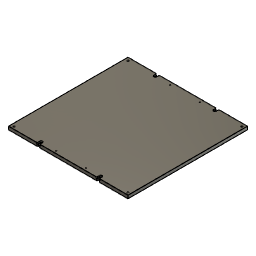
Voron_V2.4_300x300_BuildPlate (Autodesk Fusion 360 design; units mm, degrees)
Autodesk Fusion 360 part; units mm, degrees
sketch "Sketch1" plane through (0, 0, 0) normal (0, 1, 0) x (1, 0, 0)
  line L0 (0, 0) -> (300.8, 0)
  line L1 (300.8, 0) -> (300.8, 300.8)
  line L2 (300.8, 300.8) -> (0, 300.8)
  line L3 (0, 300.8) -> (0, 0)
  line L4 (0, 0) -> (7, 0)
  line L5 (7, 0) -> (7, 7) construction
  line L6 (7, 7) -> (0, 7) construction
  line L7 (0, 7) -> (0, 0)
  circle A0 centre (7, 7) radius 2.1
  line L8 (300.8, 0) -> (293.8, 0)
  line L9 (293.8, 0) -> (293.8, 7) construction
  line L10 (293.8, 7) -> (300.8, 7) construction
  line L11 (300.8, 7) -> (300.8, 0)
  circle A1 centre (293.8, 7) radius 2.1
  line L12 (150.4, 0) -> (150.4, 7) construction
  line L13 (150.4, 7) -> (75.4, 7) construction
  circle A2 centre (75.4, 7) radius 1.7
  circle A3 centre (75.4, 7) radius 3.25
  circle A4 centre (225.4, 7) radius 3.25
  circle A5 centre (225.4, 7) radius 1.7
  line L14 (300.8, 150.4) -> (290.8, 150.4) construction
  circle A6 centre (225.4, 293.8) radius 3.25
  circle A7 centre (225.4, 293.8) radius 1.7
  circle A8 centre (75.4, 293.8) radius 3.25
  circle A9 centre (75.4, 293.8) radius 1.7
  dimension "d1" = 300.8
  dimension "d2" = 300.8
  dimension "d3" = 7
  dimension "d4" = 7
  dimension "d5" = 4.2
  dimension "d6" = 7
  dimension "d7" = 7
  dimension "d8" = 4.2
  dimension "d9" = 7
  dimension "d10" = 75
  dimension "d11" = 3.4
  dimension "d12" = 6.5
  dimension "d13" = 10
  constraint horizontal L0
  constraint vertical L1
  constraint horizontal L2
  constraint vertical L3
  constraint coincident L0.start L3.end
  constraint horizontal L4
  constraint vertical L5
  constraint horizontal L6
  constraint vertical L7
  constraint coincident L5.end L6.start
  constraint horizontal L8
  constraint vertical L9
  constraint horizontal L10
  constraint vertical L11
  constraint coincident L9.end L10.start
  constraint midpoint L0 L12.start
  constraint vertical L12
  constraint perpendicular L12 L13
  constraint coincident L13.end A2.centre
  constraint concentric A2 A3
  constraint symmetric L12 A2 A5
  constraint symmetric L12 A3 A4
  constraint midpoint L1 L14.start
  constraint horizontal L14
  constraint symmetric A2 L14 A9
  constraint symmetric A3 L14 A8
  constraint symmetric A4 L14 A6
  constraint symmetric A5 L14 A7
  measures "d1" distance of L0.start L0.end
  measures "d2" distance of L0.start L2.end
  measures "d3" distance of L0.start L4.end
  measures "d4" distance of L0.start L6.end
  measures "d5" diameter of A0
  measures "d6" distance of L0.end L8.end
  measures "d7" distance of L0.end L10.end
  measures "d8" diameter of A1
  measures "d9" distance of L12.start L12.end
  measures "d10" distance of L12.end L13.end
  measures "d11" diameter of A2
  measures "d12" diameter of A3
  measures "d13" distance of L14.start L14.end
extrude "Extrude1" add sketch "Sketch1" along normal blind 8 contours L0 L1 L2 L3 L4 L7 L8 L11 | A0 | A1 | A3 | A4 | A6 | A8 makes body 1
extrude "Extrude2" cut sketch "Sketch1" along normal blind 6 contours A0 | A1 bodies 1
extrude "Extrude3" cut sketch "Sketch1" along normal blind 75 and the other way blind -4.5 contours A3 | A4 | A6 | A8 bodies 1
copy_body "Body->Comp1" bodies 1 removing the originals makes body 2 in component "Component"
chamfer "Chamfer1" distance 0.2 angle 45 8 edges at (300.8, 8, -150.4) (150.4, 8, 0) (0, 8, -150.4) (150.4, 8, -300.8) (0, 0, -150.4) (150.4, 0, 0) (300.8, 0, -150.4) (150.4, 0, -300.8) on bodies 2 in component "Component"
fillet "Fillet1" radius 0.2 4 edges at (300.8, 4, -300.8) (0, 4, -300.8) (0, 4, 0) (300.8, 4, 0) on bodies 2 in component "Component"
thread "Thread1" "ISO Metric profile 5.0 M5x0.8 6H" major diameter 5.12 minor diameter 4.234 pitch 0.8 angle 60 resizes the face on face at (9.0974, 4, -6.8953) on face at (294.6637, 4, -8.9142) on bodies 2 in component "Component"
delete_face "DeleteFace1" 1 faces at (300.7333, 7.8667, -200.4667) on bodies 2 in component "Component"
delete_face "DeleteFace2" 1 faces at (200.5333, 7.9333, -0.1333) on bodies 2 in component "Component"
delete_face "DeleteFace3" 1 faces at (200.4667, 0.1333, -0.0667) on bodies 2 in component "Component"
delete_face "DeleteFace4" 1 faces at (300.6667, 0.0667, -100.2667) on bodies 2 in component "Component"
delete_face "DeleteFace5" 1 faces at (200.5333, 0.0667, -300.6667) on bodies 2 in component "Component"
delete_face "DeleteFace6" 1 faces at (200.5333, 7.9333, -300.6667) on bodies 2 in component "Component"
delete_face "DeleteFace7" 1 faces at (0.1333, 7.9333, -200.4667) on bodies 2 in component "Component"
delete_face "DeleteFace8" 1 faces at (0.1333, 0.0667, -100.3333) on bodies 2 in component "Component"
delete_face "DeleteFace9" 1 faces at (295.0358, 4, -8.7189) on bodies 2 in component "Component"
delete_face "DeleteFace10" 1 faces at (9.1144, 2, -7.1055) on bodies 2 in component "Component"
sketch "Sketch3" plane through (0, 8, 0) normal (0, 1, 0) x (-1, 0, 0)
  circle A0 centre (-75.4, -293.8) radius 3.25
  circle A1 centre (-225.4, -7) radius 3.25
  circle A2 centre (-225.4, -293.8) radius 3.25
  circle A3 centre (-75.4, -7) radius 3.25
  arc A4 (0, -0.2) -> (-0.2, 0) centre (-0.2, -0.2) ccw
  line L0 (-0.2, 0) -> (-300.6, 0)
  arc A5 (-300.6, 0) -> (-300.8, -0.2) centre (-300.6, -0.2) ccw
  line L1 (-300.8, -0.2) -> (-300.8, -300.6)
  arc A6 (-300.8, -300.6) -> (-300.6, -300.8) centre (-300.6, -300.6) ccw
  line L2 (-300.6, -300.8) -> (-0.2, -300.8)
  arc A7 (-0.2, -300.8) -> (0, -300.6) centre (-0.2, -300.6) ccw
  line L3 (0, -300.6) -> (0, -0.2)
  line L4 (-225.4, -7) -> (-228.65, -7) construction
  line L5 (-225.4, -7) -> (-222.15, -7) construction
  line L6 (-228.65, -7) -> (-228.65, 0)
  line L7 (-222.15, -7) -> (-222.15, 0)
  constraint coincident A1.centre L4.start
  constraint coincident A1 L4.end
  constraint horizontal L4
  constraint coincident A1 L5.end
  constraint parallel L4 L5
  constraint coincident L0 L6.end
  constraint tangent A1 L6
  constraint coincident L0 L7.end
  constraint tangent A1 L7
extrude "Extrude1'" cut sketch "Sketch3" against normal blind 3.5 contours A1 L0 L6 L7 bodies 2 in component "Component"
sketch "Sketch4" plane through (0, 4.5, 0) normal (0, 1, 0) x (-1, 0, 0)
  circle A0 centre (-225.4, -7) radius 1.7
  arc A1 (-228.65, -7) -> (-222.15, -7) centre (-225.4, -7) ccw
  line L0 (-222.15, -7) -> (-222.15, 0)
  line L1 (-222.15, 0) -> (-228.65, 0)
  line L2 (-228.65, 0) -> (-228.65, -7)
  line L3 (-225.4, -7) -> (-227.1, -7) construction
  line L4 (-225.4, -7) -> (-223.7, -7) construction
  line L5 (-227.1, -7) -> (-227.1, 0)
  line L6 (-223.7, -7) -> (-223.7, 0)
  constraint coincident A0.centre A1.centre
  constraint coincident A0 L3.end
  constraint horizontal L3
  constraint coincident A0 L4.end
  constraint horizontal L4
  constraint coincident L1 L5.end
  constraint tangent A0 L5
  constraint coincident L1 L6.end
  constraint tangent A0 L6
extrude "Extrude2'" cut sketch "Sketch4" against normal blind 12 contours A0 L1 L5 L6 bodies 2 in component "Component"
fillet "Fillet2" radius 2 4 edges at (228.65, 6.25, 0) (227.1, 2.25, 0) (223.7, 2.25, 0) (222.15, 6.25, 0) on bodies 2 in component "Component"
ref_plane "WorkPlane1" through (110.95, 4, -150.4) normal (0, 0, 1) x (1, 0, 0)
mirror "Mirror1" about plane through (110.95, 4, -150.4) normal (0, 0, 1) of 11 faces at (230.1785, 6.8333, -0.0564) (228.65, 5.6667, -3.6667) (228.6339, 6.8333, -7.3236) (222.6667, 4.5, -5.3333) (223.7084, 1.5, -7.1693) (227.1, 3, -5.3333) (228.9099, 1.5, -0.0091) (222.0785, 1.5, -0.0361) (223.7, 3, -5.3333) (222.15, 6.8333, -5.3333) (220.6215, 5.6667, -0.0564) on bodies 2 in component "Component"
ref_plane "WorkPlane2" through (150.4, 4, -150.4) normal (1, 0, 0) x (0, 0, -1)
mirror "Mirror2" about plane through (150.4, 4, -150.4) normal (1, 0, 0) of 22 faces at (220.6215, 5.6667, -0.0564) (222.15, 6.8333, -5.3333) (228.6339, 6.8333, -7.3236) (222.6667, 4.5, -5.3333) (222.0785, 1.5, -0.0361) (223.7, 3, -5.3333) (223.7084, 1.5, -7.1693) (227.1, 3, -5.3333) (228.9099, 1.5, -0.0091) (228.65, 5.6667, -3.6667) (230.1785, 6.8333, -0.0564) (222.0785, 1.5, -300.7639) (223.7, 3, -295.4667) (223.7526, 3, -293.3805) (222.4052, 6.8333, -292.5376) (222.15, 6.8333, -295.4667) (220.6215, 5.6667, -300.7436) (222.6667, 4.5, -295.4667) (228.9099, 1.5, -300.7909) (227.1, 3, -295.4667) (228.65, 6.8333, -295.4667) (230.2715, 5.6667, -300.7639) on bodies 2 in component "Component"
chamfer "Chamfer4" distance 0.2 angle 45 64 edges at (221.5642, 8, -0.5858) (222.15, 8, -4.5) (225.4, 8, -10.25) (228.65, 8, -4.5) (229.2358, 8, -0.5858) (265.625, 8, 0) (300.7414, 8, -0.0586) (300.8, 8, -150.4) (300.7414, 8, -300.7414) (265.625, 8, -300.8) (229.2358, 8, -300.2142) (228.65, 8, -296.3) (225.4, 8, -290.55) (222.15, 8, -296.3) (221.5642, 8, -300.2142) (150.4, 8, -300.8) (79.2358, 8, -300.2142) (78.65, 8, -296.3) (75.4, 8, -290.55) (72.15, 8, -296.3) (71.5642, 8, -300.2142) (35.175, 8, -300.8) (0.0586, 8, -300.7414) (0, 8, -150.4) (0.0586, 8, -0.0586) (35.175, 8, 0) (71.5642, 8, -0.5858) (72.15, 8, -4.5) (75.4, 8, -10.25) (78.65, 8, -4.5) (79.2358, 8, -0.5858) (150.4, 8, 0) (77.6858, 0, -0.5858) (77.1, 0, -4.5) (75.4, 0, -8.7) (73.7, 0, -4.5) (73.1142, 0, -0.5858) (35.95, 0, 0) (0.0586, 0, -0.0586) (0, 0, -150.4) (0.0586, 0, -300.7414) (35.95, 0, -300.8) (73.1142, 0, -300.2142) (73.7, 0, -296.3) (75.4, 0, -292.1) (77.1, 0, -296.3) (77.6858, 0, -300.2142) (150.4, 0, -300.8) (223.1142, 0, -300.2142) (223.7, 0, -296.3) (225.4, 0, -292.1) (227.1, 0, -296.3) (227.6858, 0, -300.2142) (264.85, 0, -300.8) (300.7414, 0, -300.7414) (300.8, 0, -150.4) (300.7414, 0, -0.0586) (264.85, 0, 0) (227.6858, 0, -0.5858) (227.1, 0, -4.5) (225.4, 0, -8.7) (223.7, 0, -4.5) (223.1142, 0, -0.5858) (150.4, 0, 0) on bodies 2 in component "Component"
sketch "Sketch5" plane through (0, 0, 0) normal (0, -1, 0) x (1, 0, 0)
  arc A0 (79.1, -0.2) -> (77.3, -2) centre (79.1, -2) ccw
  line L0 (77.3, -2) -> (77.3, -7)
  arc A1 (73.5, -7) -> (77.3, -7) centre (75.4, -7) ccw
  line L1 (73.5, -7) -> (73.5, -2)
  arc A2 (73.5, -2) -> (71.7, -0.2) centre (71.7, -2) ccw
  line L2 (71.7, -0.2) -> (0.2, -0.2)
  line L3 (0.2, -0.2) -> (0.2, -300.6)
  line L4 (0.2, -300.6) -> (71.7, -300.6)
  arc A3 (71.7, -300.6) -> (73.5, -298.8) centre (71.7, -298.8) ccw
  line L5 (73.5, -298.8) -> (73.5, -293.8)
  arc A4 (77.3, -293.8) -> (73.5, -293.8) centre (75.4, -293.8) ccw
  line L6 (77.3, -293.8) -> (77.3, -298.8)
  arc A5 (77.3, -298.8) -> (79.1, -300.6) centre (79.1, -298.8) ccw
  line L7 (79.1, -300.6) -> (221.7, -300.6)
  arc A6 (221.7, -300.6) -> (223.5, -298.8) centre (221.7, -298.8) ccw
  line L8 (223.5, -298.8) -> (223.5, -293.8)
  arc A7 (227.3, -293.8) -> (223.5, -293.8) centre (225.4, -293.8) ccw
  line L9 (227.3, -293.8) -> (227.3, -298.8)
  arc A8 (227.3, -298.8) -> (229.1, -300.6) centre (229.1, -298.8) ccw
  line L10 (229.1, -300.6) -> (300.6, -300.6)
  line L11 (300.6, -300.6) -> (300.6, -0.2)
  line L12 (300.6, -0.2) -> (229.1, -0.2)
  arc A9 (229.1, -0.2) -> (227.3, -2) centre (229.1, -2) ccw
  line L13 (227.3, -2) -> (227.3, -7)
  arc A10 (223.5, -7) -> (227.3, -7) centre (225.4, -7) ccw
  line L14 (223.5, -7) -> (223.5, -2)
  arc A11 (223.5, -2) -> (221.7, -0.2) centre (221.7, -2) ccw
  line L15 (221.7, -0.2) -> (79.1, -0.2)
  line L16 (0, -0.2) -> (0, -300.6)
  line L17 (0.2, -300.8) -> (71.7, -300.8)
  line L18 (0, -293.8) -> (7, -293.8) construction
  line L19 (7, -293.8) -> (7, -300.8) construction
  circle A12 centre (7, -293.8) radius 2.1
  line L20 (79.1, -300.8) -> (221.7, -300.8)
  line L21 (150.4, -300.8) -> (150.4, 0) construction
  line L22 (150.4, -300.8) -> (150.4, -293.8) construction
  line L23 (150.4, -293.8) -> (112.9, -293.8) construction
  circle A13 centre (112.9, -293.8) radius 1.25
  circle A14 centre (293.8, -293.8) radius 2.1
  circle A15 centre (187.9, -293.8) radius 1.25
  line L24 (79.1, -0.2) -> (221.7, -0.2)
  line L25 (221.7, 0) -> (79.1, 0)
  line L26 (150.4, -150.4) -> (231.0911, -150.4) construction
  circle A16 centre (7, -7) radius 2.1
  circle A17 centre (112.9, -7) radius 1.25
  circle A18 centre (187.9, -7) radius 1.25
  circle A19 centre (293.8, -7) radius 2.1
  dimension "d36" = 7
  dimension "d37" = 7
  dimension "d38" = 4.2
  dimension "d39" = 7
  dimension "d40" = 37.5
  dimension "d41" = 2.5
  constraint coincident L16 L18.start
  constraint perpendicular L3 L18
  constraint coincident L17 L19.end
  constraint perpendicular L17 L19
  constraint coincident L18.end L19.start
  constraint midpoint L20 L21.start
  constraint perpendicular L15 L21
  constraint perpendicular L7 L22
  constraint perpendicular L22 L23
  constraint coincident L23.end A13.centre
  constraint symmetric A12 L21 A14
  constraint symmetric L21 A13 A15
  constraint coincident L25 L21.end
  constraint midpoint L21 L26.start
  constraint perpendicular L21 L26
  constraint symmetric A12 L26 A16
  constraint symmetric A13 L26 A17
  constraint symmetric A14 L26 A19
  constraint symmetric A15 L26 A18
  measures "d36" distance of L18.start L18.end
  measures "d37" distance of L18.end L19.end
  measures "d38" diameter of A12
  measures "d39" distance of L21.start L22.end
  measures "d40" distance of L22.end L23.end
  measures "d41" diameter of A13
extrude "Extrude3'" cut sketch "Sketch5" against normal blind 7 contours A12 | A13 | A14 | A15 | A16 | A17 | A18 | A19 bodies 2 in component "Component"
chamfer "Chamfer2" [suppressed] in component "Component"
chamfer "Chamfer3" [suppressed] in component "Component"
component "Component" placed x (1, 0, 0) y (0, 1, 0) z (0, 0, 1) at (0, 0, 0)
equation "d20 = -8.00 mm + 3.5 mm"
equation "d40 = ( 75 / 2 ) * 1 mm"
